Autodesk Fusion 360 part; units mm, degrees
(part 2 of 6)
  spline S10 degree 5 poles (8.3108, -19.4412) (8.3159, -19.4531) (8.3264, -19.4767) (8.3432, -19.5116) (8.3675, -19.5571) (8.4005, -19.6127) (8.4354, -19.6674) (8.4715, -19.7215) (8.5082, -19.7752) (8.5453, -19.8288) (8.583, -19.8822) (8.6212, -19.9352) (8.6602, -19.9878) (8.7001, -20.0399) (8.7409, -20.0915) (8.7826, -20.1426) (8.825, -20.1933) (8.868, -20.2437) (8.9115, -20.2938) (8.9555, -20.3436) (9, -20.3931) (9.045, -20.4423) (9.0905, -20.4911) (9.1367, -20.5396) (9.1833, -20.5878) (9.2305, -20.6356) (9.2782, -20.6831) (9.3264, -20.7304) (9.375, -20.7773) (9.424, -20.8239) (9.4735, -20.8702) (9.5235, -20.9163) (9.5738, -20.962) (9.6246, -21.0074) (9.6759, -21.0526) (9.7275, -21.0974) (9.7796, -21.142) (9.8321, -21.1862) (9.885, -21.2302) (9.9382, -21.2739) (9.9919, -21.3173) (10.0459, -21.3605) (10.1003, -21.4033) (10.155, -21.4459) (10.2102, -21.4882) (10.2657, -21.5302) (10.3216, -21.5719) (10.3778, -21.6133) (10.4343, -21.6545) (10.4913, -21.6954) (10.5485, -21.736) (10.6061, -21.7763) (10.664, -21.8163) (10.7223, -21.8561) (10.7809, -21.8956) (10.8398, -21.9348) (10.899, -21.9738) (10.9586, -22.0124) (11.0184, -22.0508) (11.0786, -22.0889) (11.1391, -22.1268) (11.1999, -22.1643) (11.261, -22.2016) (11.3224, -22.2386) (11.3841, -22.2754) (11.4461, -22.3119) (11.5083, -22.348) (11.5709, -22.384) (11.6337, -22.4196) (11.6969, -22.455) (11.7603, -22.4901) (11.8112, -22.5179) (11.8496, -22.5387) (11.8752, -22.5525) (11.888, -22.5594) knots 0 0 0 0 0 0 0.01428571 0.02857143 0.04285714 0.05714286 0.07142857 0.08571429 0.1 0.11428571 0.12857143 0.14285714 0.15714286 0.17142857 0.18571429 0.2 0.21428571 0.22857143 0.24285714 0.25714286 0.27142857 0.28571429 0.3 0.31428571 0.32857143 0.34285714 0.35714286 0.37142857 0.38571429 0.4 0.41428571 0.42857143 0.44285714 0.45714286 0.47142857 0.48571429 0.5 0.51428571 0.52857143 0.54285714 0.55714286 0.57142857 0.58571429 0.6 0.61428571 0.62857143 0.64285714 0.65714286 0.67142857 0.68571429 0.7 0.71428571 0.72857143 0.74285714 0.75714286 0.77142857 0.78571429 0.8 0.81428571 0.82857143 0.84285714 0.85714286 0.87142857 0.88571429 0.9 0.91428571 0.92857143 0.94285714 0.95714286 0.97142857 0.98571429 1 1 1 1 1 1
  arc A22 (11.888, -22.5594) -> (13.593, -21.575) centre (0, 0) ccw
  spline S11 degree 5 poles (13.593, -21.575) (13.5934, -21.5605) (13.5943, -21.5314) (13.5955, -21.4878) (13.5968, -21.4297) (13.5981, -21.3573) (13.5991, -21.2849) (13.5996, -21.2127) (13.5998, -21.1405) (13.5996, -21.0685) (13.599, -20.9966) (13.598, -20.9248) (13.5967, -20.8531) (13.5949, -20.7816) (13.5928, -20.7101) (13.5903, -20.6388) (13.5874, -20.5677) (13.584, -20.4966) (13.5803, -20.4257) (13.5762, -20.3549) (13.5717, -20.2843) (13.5668, -20.2138) (13.5615, -20.1435) (13.5558, -20.0733) (13.5496, -20.0033) (13.5431, -19.9334) (13.5362, -19.8636) (13.5288, -19.7941) (13.521, -19.7247) (13.5128, -19.6554) (13.5042, -19.5864) (13.4952, -19.5175) (13.4857, -19.4488) (13.4758, -19.3802) (13.4654, -19.3119) (13.4547, -19.2437) (13.4434, -19.1757) (13.4318, -19.108) (13.4197, -19.0404) (13.4071, -18.973) (13.3941, -18.9059) (13.3807, -18.8389) (13.3667, -18.7722) (13.3523, -18.7057) (13.3374, -18.6394) (13.322, -18.5734) (13.3062, -18.5076) (13.2898, -18.442) (13.273, -18.3767) (13.2557, -18.3117) (13.2379, -18.2469) (13.2195, -18.1824) (13.2006, -18.1182) (13.181, -18.0543) (13.1609, -17.9908) (13.1403, -17.9275) (13.1192, -17.8645) (13.0976, -17.8018) (13.0754, -17.7393) (13.0527, -17.6773) (13.0293, -17.6156) (13.005, -17.5545) (12.9798, -17.4938) (12.9538, -17.4338) (12.927, -17.3741) (12.8996, -17.3149) (12.8718, -17.2559) (12.8435, -17.1973) (12.8147, -17.139) (12.7848, -17.0814) (12.7532, -17.025) (12.7259, -16.9812) (12.7041, -16.9492) (12.6889, -16.9283) (12.6811, -16.918) knots -1 -1 -1 -1 -1 -1 -0.98571429 -0.97142857 -0.95714286 -0.94285714 -0.92857143 -0.91428571 -0.9 -0.88571429 -0.87142857 -0.85714286 -0.84285714 -0.82857143 -0.81428571 -0.8 -0.78571429 -0.77142857 -0.75714286 -0.74285714 -0.72857143 -0.71428571 -0.7 -0.68571429 -0.67142857 -0.65714286 -0.64285714 -0.62857143 -0.61428571 -0.6 -0.58571429 -0.57142857 -0.55714286 -0.54285714 -0.52857143 -0.51428571 -0.5 -0.48571429 -0.47142857 -0.45714286 -0.44285714 -0.42857143 -0.41428571 -0.4 -0.38571429 -0.37142857 -0.35714286 -0.34285714 -0.32857143 -0.31428571 -0.3 -0.28571429 -0.27142857 -0.25714286 -0.24285714 -0.22857143 -0.21428571 -0.2 -0.18571429 -0.17142857 -0.15714286 -0.14285714 -0.12857143 -0.11428571 -0.1 -0.08571429 -0.07142857 -0.05714286 -0.04285714 -0.02857143 -0.01428571 0 0 0 0 0 0
  line L11 (12.6811, -16.918) -> (12.1717, -16.2376)
  arc A23 (12.3867, -14.2079) -> (12.1717, -16.2376) centre (13.3724, -15.3385) ccw
  arc A24 (12.3867, -14.2079) -> (12.8353, -13.8039) centre (0, 0) ccw
  arc A25 (14.8763, -13.8023) -> (12.8353, -13.8039) centre (13.8567, -14.9024) ccw
  line L12 (14.8763, -13.8023) -> (15.4998, -14.3801)
  spline S12 degree 5 poles (15.4998, -14.3801) (15.5093, -14.3889) (15.5285, -14.4062) (15.558, -14.4312) (15.5987, -14.4629) (15.6515, -14.5003) (15.7056, -14.536) (15.7605, -14.5708) (15.8159, -14.605) (15.8717, -14.6388) (15.9277, -14.6723) (15.9842, -14.7051) (16.0412, -14.7373) (16.0989, -14.7687) (16.1572, -14.7992) (16.2161, -14.829) (16.2754, -14.8581) (16.3352, -14.8866) (16.3953, -14.9147) (16.4557, -14.9423) (16.5165, -14.9694) (16.5776, -14.996) (16.6391, -15.0221) (16.701, -15.0477) (16.7632, -15.0727) (16.8258, -15.0972) (16.8886, -15.1212) (16.9518, -15.1447) (17.0153, -15.1678) (17.0791, -15.1905) (17.1432, -15.2127) (17.2075, -15.2344) (17.2721, -15.2557) (17.337, -15.2766) (17.4022, -15.297) (17.4676, -15.3169) (17.5333, -15.3364) (17.5993, -15.3555) (17.6655, -15.3742) (17.7319, -15.3925) (17.7986, -15.4103) (17.8655, -15.4277) (17.9326, -15.4448) (17.9999, -15.4614) (18.0675, -15.4776) (18.1353, -15.4934) (18.2033, -15.5087) (18.2715, -15.5237) (18.3399, -15.5383) (18.4085, -15.5525) (18.4774, -15.5663) (18.5464, -15.5797) (18.6156, -15.5928) (18.685, -15.6054) (18.7546, -15.6177) (18.8243, -15.6295) (18.8943, -15.641) (18.9644, -15.6521) (19.0347, -15.6628) (19.1052, -15.6732) (19.1758, -15.6831) (19.2467, -15.6927) (19.3176, -15.7019) (19.3888, -15.7108) (19.4601, -15.7193) (19.5315, -15.7274) (19.6032, -15.7351) (19.6749, -15.7425) (19.7468, -15.7495) (19.8189, -15.7561) (19.8911, -15.7624) (19.949, -15.7671) (19.9924, -15.7705) (20.0215, -15.7726) (20.036, -15.7737) knots 0 0 0 0 0 0 0.01428571 0.02857143 0.04285714 0.05714286 0.07142857 0.08571429 0.1 0.11428571 0.12857143 0.14285714 0.15714286 0.17142857 0.18571429 0.2 0.21428571 0.22857143 0.24285714 0.25714286 0.27142857 0.28571429 0.3 0.31428571 0.32857143 0.34285714 0.35714286 0.37142857 0.38571429 0.4 0.41428571 0.42857143 0.44285714 0.45714286 0.47142857 0.48571429 0.5 0.51428571 0.52857143 0.54285714 0.55714286 0.57142857 0.58571429 0.6 0.61428571 0.62857143 0.64285714 0.65714286 0.67142857 0.68571429 0.7 0.71428571 0.72857143 0.74285714 0.75714286 0.77142857 0.78571429 0.8 0.81428571 0.82857143 0.84285714 0.85714286 0.87142857 0.88571429 0.9 0.91428571 0.92857143 0.94285714 0.95714286 0.97142857 0.98571429 1 1 1 1 1 1
  arc A26 (20.036, -15.7737) -> (21.1931, -14.181) centre (0, 0) ccw
  spline S13 degree 5 poles (21.1931, -14.181) (21.1876, -14.1675) (21.1766, -14.1406) (21.16, -14.1003) (21.1376, -14.0467) (21.1093, -13.98) (21.0807, -13.9135) (21.0519, -13.8473) (21.0227, -13.7813) (20.9932, -13.7156) (20.9634, -13.6501) (20.9333, -13.5849) (20.9029, -13.52) (20.8722, -13.4553) (20.8412, -13.391) (20.8099, -13.3268) (20.7783, -13.263) (20.7464, -13.1995) (20.7141, -13.1362) (20.6816, -13.0732) (20.6488, -13.0105) (20.6156, -12.9481) (20.5821, -12.886) (20.5484, -12.8242) (20.5143, -12.7627) (20.4799, -12.7016) (20.4452, -12.6407) (20.4101, -12.5801) (20.3748, -12.5199) (20.3392, -12.46) (20.3032, -12.4004) (20.2669, -12.3411) (20.2303, -12.2822) (20.1934, -12.2236) (20.1561, -12.1654) (20.1186, -12.1075) (20.0807, -12.05) (20.0425, -11.9928) (20.0039, -11.936) (19.965, -11.8795) (19.9258, -11.8235) (19.8863, -11.7678) (19.8464, -11.7125) (19.8062, -11.6576) (19.7656, -11.6032) (19.7247, -11.5491) (19.6835, -11.4954) (19.6419, -11.4422) (19.6, -11.3893) (19.5577, -11.337) (19.5151, -11.285) (19.4721, -11.2336) (19.4286, -11.1826) (19.3848, -11.1322) (19.3406, -11.0823) (19.2961, -11.0329) (19.2511, -10.984) (19.2059, -10.9355) (19.1603, -10.8874) (19.1142, -10.84) (19.0677, -10.7932) (19.0207, -10.7472) (18.973, -10.702) (18.9248, -10.6577) (18.8761, -10.6142) (18.827, -10.5712) (18.7776, -10.5287) (18.7279, -10.4865) (18.6779, -10.445) (18.6272, -10.4046) (18.5753, -10.366) (18.5326, -10.337) (18.4996, -10.3167) (18.4773, -10.3038) (18.466, -10.2975) knots -1 -1 -1 -1 -1 -1 -0.98571429 -0.97142857 -0.95714286 -0.94285714 -0.92857143 -0.91428571 -0.9 -0.88571429 -0.87142857 -0.85714286 -0.84285714 -0.82857143 -0.81428571 -0.8 -0.78571429 -0.77142857 -0.75714286 -0.74285714 -0.72857143 -0.71428571 -0.7 -0.68571429 -0.67142857 -0.65714286 -0.64285714 -0.62857143 -0.61428571 -0.6 -0.58571429 -0.57142857 -0.55714286 -0.54285714 -0.52857143 -0.51428571 -0.5 -0.48571429 -0.47142857 -0.45714286 -0.44285714 -0.42857143 -0.41428571 -0.4 -0.38571429 -0.37142857 -0.35714286 -0.34285714 -0.32857143 -0.31428571 -0.3 -0.28571429 -0.27142857 -0.25714286 -0.24285714 -0.22857143 -0.21428571 -0.2 -0.18571429 -0.17142857 -0.15714286 -0.14285714 -0.12857143 -0.11428571 -0.1 -0.08571429 -0.07142857 -0.05714286 -0.04285714 -0.02857143 -0.01428571 0 0 0 0 0 0
  line L13 (18.466, -10.2975) -> (17.7238, -9.8831)
  arc A27 (17.0946, -7.9414) -> (17.7238, -9.8831) centre (18.455, -8.5734) ccw
  arc A28 (17.0946, -7.9414) -> (17.3402, -7.3899) centre (0, 0) ccw
  arc A29 (19.2041, -6.5583) -> (17.3402, -7.3899) centre (18.7201, -7.978) ccw
  line L14 (19.2041, -6.5583) -> (20.0087, -6.8325)
  spline S14 degree 5 poles (20.0087, -6.8325) (20.0209, -6.8367) (20.0455, -6.8447) (20.0826, -6.8556) (20.1327, -6.868) (20.1961, -6.8807) (20.2601, -6.8913) (20.3244, -6.9007) (20.389, -6.9094) (20.4536, -6.9176) (20.5184, -6.9254) (20.5834, -6.9325) (20.6486, -6.9387) (20.714, -6.9438) (20.7797, -6.948) (20.8456, -6.9513) (20.9117, -6.9537) (20.9779, -6.9555) (21.0442, -6.9567) (21.1106, -6.9573) (21.1772, -6.9574) (21.2438, -6.9568) (21.3106, -6.9556) (21.3775, -6.9538) (21.4445, -6.9514) (21.5117, -6.9483) (21.5789, -6.9447) (21.6462, -6.9405) (21.7136, -6.9357) (21.7811, -6.9305) (21.8486, -6.9247) (21.9163, -6.9184) (21.9839, -6.9116) (22.0517, -6.9042) (22.1195, -6.8963) (22.1874, -6.888) (22.2554, -6.8791) (22.3234, -6.8697) (22.3915, -6.8598) (22.4596, -6.8495) (22.5277, -6.8387) (22.5959, -6.8274) (22.6642, -6.8157) (22.7324, -6.8034) (22.8008, -6.7907) (22.8691, -6.7776) (22.9375, -6.764) (23.0059, -6.7499) (23.0744, -6.7355) (23.1428, -6.7205) (23.2113, -6.7051) (23.2798, -6.6893) (23.3483, -6.6731) (23.4169, -6.6564) (23.4854, -6.6393) (23.554, -6.6217) (23.6226, -6.6038) (23.6911, -6.5854) (23.7597, -6.5666) (23.8283, -6.5474) (23.8969, -6.5277) (23.9655, -6.5077) (24.0341, -6.4873) (24.1027, -6.4664) (24.1713, -6.4451) (24.2398, -6.4235) (24.3084, -6.4014) (24.377, -6.3789) (24.4455, -6.3561) (24.514, -6.3328) (24.5825, -6.3092) (24.6373, -6.29) (24.6784, -6.2754) (24.7058, -6.2656) (24.7195, -6.2606) knots 0 0 0 0 0 0 0.01428571 0.02857143 0.04285714 0.05714286 0.07142857 0.08571429 0.1 0.11428571 0.12857143 0.14285714 0.15714286 0.17142857 0.18571429 0.2 0.21428571 0.22857143 0.24285714 0.25714286 0.27142857 0.28571429 0.3 0.31428571 0.32857143 0.34285714 0.35714286 0.37142857 0.38571429 0.4 0.41428571 0.42857143 0.44285714 0.45714286 0.47142857 0.48571429 0.5 0.51428571 0.52857143 0.54285714 0.55714286 0.57142857 0.58571429 0.6 0.61428571 0.62857143 0.64285714 0.65714286 0.67142857 0.68571429 0.7 0.71428571 0.72857143 0.74285714 0.75714286 0.77142857 0.78571429 0.8 0.81428571 0.82857143 0.84285714 0.85714286 0.87142857 0.88571429 0.9 0.91428571 0.92857143 0.94285714 0.95714286 0.97142857 0.98571429 1 1 1 1 1 1
  arc A30 (24.7195, -6.2606) -> (25.1288, -4.335) centre (0, 0) ccw
  spline S15 degree 5 poles (25.1288, -4.335) (25.1183, -4.3249) (25.0973, -4.3048) (25.0657, -4.2747) (25.0234, -4.2349) (24.9705, -4.1854) (24.9173, -4.1363) (24.864, -4.0875) (24.8105, -4.0391) (24.7569, -3.9911) (24.703, -3.9434) (24.649, -3.8961) (24.5948, -3.8491) (24.5405, -3.8026) (24.486, -3.7564) (24.4313, -3.7105) (24.3765, -3.6651) (24.3215, -3.62) (24.2663, -3.5753) (24.2109, -3.531) (24.1554, -3.4871) (24.0998, -3.4436) (24.0439, -3.4005) (23.9879, -3.3578) (23.9318, -3.3154) (23.8755, -3.2735) (23.819, -3.232) (23.7624, -3.191) (23.7056, -3.1503) (23.6487, -3.1101) (23.5916, -3.0703) (23.5343, -3.0309) (23.4769, -2.9919) (23.4194, -2.9534) (23.3617, -2.9154) (23.3038, -2.8778) (23.2458, -2.8406) (23.1876, -2.804) (23.1293, -2.7677) (23.0708, -2.732) (23.0122, -2.6967) (22.9534, -2.6619) (22.8945, -2.6276) (22.8355, -2.5939) (22.7762, -2.5606) (22.7169, -2.5278) (22.6574, -2.4956) (22.5977, -2.4639) (22.538, -2.4326) (22.478, -2.402) (22.4179, -2.3719) (22.3577, -2.3424) (22.2973, -2.3135) (22.2368, -2.2853) (22.1761, -2.2577) (22.1153, -2.2307) (22.0544, -2.2042) (21.9933, -2.1783) (21.9321, -2.153) (21.8707, -2.1284) (21.8092, -2.1045) (21.7475, -2.0816) (21.6856, -2.0598) (21.6236, -2.0389) (21.5613, -2.019) (21.499, -1.9997) (21.4366, -1.9809) (21.3741, -1.9626) (21.3115, -1.945) (21.2487, -1.9287) (21.1856, -1.9145) (21.1348, -1.9055) (21.0964, -1.9003) (21.0707, -1.8976) (21.0579, -1.8964) knots -1 -1 -1 -1 -1 -1 -0.98571429 -0.97142857 -0.95714286 -0.94285714 -0.92857143 -0.91428571 -0.9 -0.88571429 -0.87142857 -0.85714286 -0.84285714 -0.82857143 -0.81428571 -0.8 -0.78571429 -0.77142857 -0.75714286 -0.74285714 -0.72857143 -0.71428571 -0.7 -0.68571429 -0.67142857 -0.65714286 -0.64285714 -0.62857143 -0.61428571 -0.6 -0.58571429 -0.57142857 -0.55714286 -0.54285714 -0.52857143 -0.51428571 -0.5 -0.48571429 -0.47142857 -0.45714286 -0.44285714 -0.42857143 -0.41428571 -0.4 -0.38571429 -0.37142857 -0.35714286 -0.34285714 -0.32857143 -0.31428571 -0.3 -0.28571429 -0.27142857 -0.25714286 -0.24285714 -0.22857143 -0.21428571 -0.2 -0.18571429 -0.17142857 -0.15714286 -0.14285714 -0.12857143 -0.11428571 -0.1 -0.08571429 -0.07142857 -0.05714286 -0.04285714 -0.02857143 -0.01428571 0 0 0 0 0 0
  line L15 (21.0579, -1.8964) -> (20.2113, -1.8197)
  arc A31 (18.8468, -0.3018) -> (20.2113, -1.8197) centre (20.3466, -0.3259) ccw
  arc A32 (18.8468, -0.3018) -> (18.8468, 0.3018) centre (0, 0) ccw
  arc A33 (20.2113, 1.8197) -> (18.8468, 0.3018) centre (20.3466, 0.3259) ccw
  line L16 (20.2113, 1.8197) -> (21.0579, 1.8964)
  spline S16 degree 5 poles (21.0579, 1.8964) (21.0707, 1.8976) (21.0964, 1.9003) (21.1348, 1.9055) (21.1856, 1.9145) (21.2487, 1.9287) (21.3115, 1.945) (21.3741, 1.9626) (21.4366, 1.9809) (21.499, 1.9997) (21.5613, 2.019) (21.6236, 2.0389) (21.6856, 2.0598) (21.7475, 2.0816) (21.8092, 2.1045) (21.8707, 2.1284) (21.9321, 2.153) (21.9933, 2.1783) (22.0544, 2.2042) (22.1153, 2.2307) (22.1761, 2.2577) (22.2368, 2.2853) (22.2973, 2.3135) (22.3577, 2.3424) (22.4179, 2.3719) (22.478, 2.402) (22.538, 2.4326) (22.5977, 2.4639) (22.6574, 2.4956) (22.7169, 2.5278) (22.7762, 2.5606) (22.8355, 2.5939) (22.8945, 2.6276) (22.9534, 2.6619) (23.0122, 2.6967) (23.0708, 2.732) (23.1293, 2.7677) (23.1876, 2.804) (23.2458, 2.8406) (23.3038, 2.8778) (23.3617, 2.9154) (23.4194, 2.9534) (23.4769, 2.9919) (23.5343, 3.0309) (23.5916, 3.0703) (23.6487, 3.1101) (23.7056, 3.1503) (23.7624, 3.191) (23.819, 3.232) (23.8755, 3.2735) (23.9318, 3.3154) (23.9879, 3.3578) (24.0439, 3.4005) (24.0998, 3.4436) (24.1554, 3.4871) (24.2109, 3.531) (24.2663, 3.5753) (24.3215, 3.62) (24.3765, 3.6651) (24.4313, 3.7105) (24.486, 3.7564) (24.5405, 3.8026) (24.5948, 3.8491) (24.649, 3.8961) (24.703, 3.9434) (24.7569, 3.9911) (24.8105, 4.0391) (24.864, 4.0875) (24.9173, 4.1363) (24.9705, 4.1854) (25.0234, 4.2349) (25.0657, 4.2747) (25.0973, 4.3048) (25.1183, 4.3249) (25.1288, 4.335) knots 0 0 0 0 0 0 0.01428571 0.02857143 0.04285714 0.05714286 0.07142857 0.08571429 0.1 0.11428571 0.12857143 0.14285714 0.15714286 0.17142857 0.18571429 0.2 0.21428571 0.22857143 0.24285714 0.25714286 0.27142857 0.28571429 0.3 0.31428571 0.32857143 0.34285714 0.35714286 0.37142857 0.38571429 0.4 0.41428571 0.42857143 0.44285714 0.45714286 0.47142857 0.48571429 0.5 0.51428571 0.52857143 0.54285714 0.55714286 0.57142857 0.58571429 0.6 0.61428571 0.62857143 0.64285714 0.65714286 0.67142857 0.68571429 0.7 0.71428571 0.72857143 0.74285714 0.75714286 0.77142857 0.78571429 0.8 0.81428571 0.82857143 0.84285714 0.85714286 0.87142857 0.88571429 0.9 0.91428571 0.92857143 0.94285714 0.95714286 0.97142857 0.98571429 1 1 1 1 1 1
  arc A34 (25.1288, 4.335) -> (24.7195, 6.2606) centre (0, 0) ccw
  spline S17 degree 5 poles (24.7195, 6.2606) (24.7058, 6.2656) (24.6784, 6.2754) (24.6373, 6.29) (24.5825, 6.3092) (24.514, 6.3328) (24.4455, 6.3561) (24.377, 6.3789) (24.3084, 6.4014) (24.2398, 6.4235) (24.1713, 6.4451) (24.1027, 6.4664) (24.0341, 6.4873) (23.9655, 6.5077) (23.8969, 6.5277) (23.8283, 6.5474) (23.7597, 6.5666) (23.6911, 6.5854) (23.6226, 6.6038) (23.554, 6.6217) (23.4854, 6.6393) (23.4169, 6.6564) (23.3483, 6.6731) (23.2798, 6.6893) (23.2113, 6.7051) (23.1428, 6.7205) (23.0744, 6.7355) (23.0059, 6.7499) (22.9375, 6.764) (22.8691, 6.7776) (22.8008, 6.7907) (22.7324, 6.8034) (22.6642, 6.8157) (22.5959, 6.8274) (22.5277, 6.8387) (22.4596, 6.8495) (22.3915, 6.8598) (22.3234, 6.8697) (22.2554, 6.8791) (22.1874, 6.888) (22.1195, 6.8963) (22.0517, 6.9042) (21.9839, 6.9116) (21.9163, 6.9184) (21.8486, 6.9247) (21.7811, 6.9305) (21.7136, 6.9357) (21.6462, 6.9405) (21.5789, 6.9447) (21.5117, 6.9483) (21.4445, 6.9514) (21.3775, 6.9538) (21.3106, 6.9556) (21.2438, 6.9568) (21.1772, 6.9574) (21.1106, 6.9573) (21.0442, 6.9567) (20.9779, 6.9555) (20.9117, 6.9537) (20.8456, 6.9513) (20.7797, 6.948) (20.714, 6.9438) (20.6486, 6.9387) (20.5834, 6.9325) (20.5184, 6.9254) (20.4536, 6.9176) (20.389, 6.9094) (20.3244, 6.9007) (20.2601, 6.8913) (20.1961, 6.8807) (20.1327, 6.868) (20.0826, 6.8556) (20.0455, 6.8447) (20.0209, 6.8367) (20.0087, 6.8325) knots -1 -1 -1 -1 -1 -1 -0.98571429 -0.97142857 -0.95714286 -0.94285714 -0.92857143 -0.91428571 -0.9 -0.88571429 -0.87142857 -0.85714286 -0.84285714 -0.82857143 -0.81428571 -0.8 -0.78571429 -0.77142857 -0.75714286 -0.74285714 -0.72857143 -0.71428571 -0.7 -0.68571429 -0.67142857 -0.65714286 -0.64285714 -0.62857143 -0.61428571 -0.6 -0.58571429 -0.57142857 -0.55714286 -0.54285714 -0.52857143 -0.51428571 -0.5 -0.48571429 -0.47142857 -0.45714286 -0.44285714 -0.42857143 -0.41428571 -0.4 -0.38571429 -0.37142857 -0.35714286 -0.34285714 -0.32857143 -0.31428571 -0.3 -0.28571429 -0.27142857 -0.25714286 -0.24285714 -0.22857143 -0.21428571 -0.2 -0.18571429 -0.17142857 -0.15714286 -0.14285714 -0.12857143 -0.11428571 -0.1 -0.08571429 -0.07142857 -0.05714286 -0.04285714 -0.02857143 -0.01428571 0 0 0 0 0 0
  line L17 (20.0087, 6.8325) -> (19.2041, 6.5583)
  arc A35 (17.3402, 7.3899) -> (19.2041, 6.5583) centre (18.7201, 7.978) ccw
  arc A36 (17.3402, 7.3899) -> (17.0946, 7.9414) centre (0, 0) ccw
  arc A37 (17.7238, 9.8831) -> (17.0946, 7.9414) centre (18.455, 8.5734) ccw
  line L18 (17.7238, 9.8831) -> (18.466, 10.2975)
  spline S18 degree 5 poles (18.466, 10.2975) (18.4773, 10.3038) (18.4996, 10.3167) (18.5326, 10.337) (18.5753, 10.366) (18.6272, 10.4046) (18.6779, 10.445) (18.7279, 10.4865) (18.7776, 10.5287) (18.827, 10.5712) (18.8761, 10.6142) (18.9248, 10.6577) (18.973, 10.702) (19.0207, 10.7472) (19.0677, 10.7932) (19.1142, 10.84) (19.1603, 10.8874) (19.2059, 10.9355) (19.2511, 10.984) (19.2961, 11.0329) (19.3406, 11.0823) (19.3848, 11.1322) (19.4286, 11.1826) (19.4721, 11.2336) (19.5151, 11.285) (19.5577, 11.337) (19.6, 11.3893) (19.6419, 11.4422) (19.6835, 11.4954) (19.7247, 11.5491) (19.7656, 11.6032) (19.8062, 11.6576) (19.8464, 11.7125) (19.8863, 11.7678) (19.9258, 11.8235) (19.965, 11.8795) (20.0039, 11.936) (20.0425, 11.9928) (20.0807, 12.05) (20.1186, 12.1075) (20.1561, 12.1654) (20.1934, 12.2236) (20.2303, 12.2822) (20.2669, 12.3411) (20.3032, 12.4004) (20.3392, 12.46) (20.3748, 12.5199) (20.4101, 12.5801) (20.4452, 12.6407) (20.4799, 12.7016) (20.5143, 12.7627) (20.5484, 12.8242) (20.5821, 12.886) (20.6156, 12.9481) (20.6488, 13.0105) (20.6816, 13.0732) (20.7141, 13.1362) (20.7464, 13.1995) (20.7783, 13.263) (20.8099, 13.3268) (20.8412, 13.391) (20.8722, 13.4553) (20.9029, 13.52) (20.9333, 13.5849) (20.9634, 13.6501) (20.9932, 13.7156) (21.0227, 13.7813) (21.0519, 13.8473) (21.0807, 13.9135) (21.1093, 13.98) (21.1376, 14.0467) (21.16, 14.1003) (21.1766, 14.1406) (21.1876, 14.1675) (21.1931, 14.181) knots 0 0 0 0 0 0 0.01428571 0.02857143 0.04285714 0.05714286 0.07142857 0.08571429 0.1 0.11428571 0.12857143 0.14285714 0.15714286 0.17142857 0.18571429 0.2 0.21428571 0.22857143 0.24285714 0.25714286 0.27142857 0.28571429 0.3 0.31428571 0.32857143 0.34285714 0.35714286 0.37142857 0.38571429 0.4 0.41428571 0.42857143 0.44285714 0.45714286 0.47142857 0.48571429 0.5 0.51428571 0.52857143 0.54285714 0.55714286 0.57142857 0.58571429 0.6 0.61428571 0.62857143 0.64285714 0.65714286 0.67142857 0.68571429 0.7 0.71428571 0.72857143 0.74285714 0.75714286 0.77142857 0.78571429 0.8 0.81428571 0.82857143 0.84285714 0.85714286 0.87142857 0.88571429 0.9 0.91428571 0.92857143 0.94285714 0.95714286 0.97142857 0.98571429 1 1 1 1 1 1
  arc A38 (21.1931, 14.181) -> (20.036, 15.7737) centre (0, 0) ccw
  spline S19 degree 5 poles (20.036, 15.7737) (20.0215, 15.7726) (19.9924, 15.7705) (19.949, 15.7671) (19.8911, 15.7624) (19.8189, 15.7561) (19.7468, 15.7495) (19.6749, 15.7425) (19.6032, 15.7351) (19.5315, 15.7274) (19.4601, 15.7193) (19.3888, 15.7108) (19.3176, 15.7019) (19.2467, 15.6927) (19.1758, 15.6831) (19.1052, 15.6732) (19.0347, 15.6628) (18.9644, 15.6521) (18.8943, 15.641) (18.8243, 15.6295) (18.7546, 15.6177) (18.685, 15.6054) (18.6156, 15.5928) (18.5464, 15.5797) (18.4774, 15.5663) (18.4085, 15.5525) (18.3399, 15.5383) (18.2715, 15.5237) (18.2033, 15.5087) (18.1353, 15.4934) (18.0675, 15.4776) (17.9999, 15.4614) (17.9326, 15.4448) (17.8655, 15.4277) (17.7986, 15.4103) (17.7319, 15.3925) (17.6655, 15.3742) (17.5993, 15.3555) (17.5333, 15.3364) (17.4676, 15.3169) (17.4022, 15.297) (17.337, 15.2766) (17.2721, 15.2557) (17.2075, 15.2344) (17.1432, 15.2127) (17.0791, 15.1905) (17.0153, 15.1678) (16.9518, 15.1447) (16.8886, 15.1212) (16.8258, 15.0972) (16.7632, 15.0727) (16.701, 15.0477) (16.6391, 15.0221) (16.5776, 14.996) (16.5165, 14.9694) (16.4557, 14.9423) (16.3953, 14.9147) (16.3352, 14.8866) (16.2754, 14.8581) (16.2161, 14.829) (16.1572, 14.7992) (16.0989, 14.7687) (16.0412, 14.7373) (15.9842, 14.7051) (15.9277, 14.6723) (15.8717, 14.6388) (15.8159, 14.605) (15.7605, 14.5708) (15.7056, 14.536) (15.6515, 14.5003) (15.5987, 14.4629) (15.558, 14.4312) (15.5285, 14.4062) (15.5093, 14.3889) (15.4998, 14.3801) knots -1 -1 -1 -1 -1 -1 -0.98571429 -0.97142857 -0.95714286 -0.94285714 -0.92857143 -0.91428571 -0.9 -0.88571429 -0.87142857 -0.85714286 -0.84285714 -0.82857143 -0.81428571 -0.8 -0.78571429 -0.77142857 -0.75714286 -0.74285714 -0.72857143 -0.71428571 -0.7 -0.68571429 -0.67142857 -0.65714286 -0.64285714 -0.62857143 -0.61428571 -0.6 -0.58571429 -0.57142857 -0.55714286 -0.54285714 -0.52857143 -0.51428571 -0.5 -0.48571429 -0.47142857 -0.45714286 -0.44285714 -0.42857143 -0.41428571 -0.4 -0.38571429 -0.37142857 -0.35714286 -0.34285714 -0.32857143 -0.31428571 -0.3 -0.28571429 -0.27142857 -0.25714286 -0.24285714 -0.22857143 -0.21428571 -0.2 -0.18571429 -0.17142857 -0.15714286 -0.14285714 -0.12857143 -0.11428571 -0.1 -0.08571429 -0.07142857 -0.05714286 -0.04285714 -0.02857143 -0.01428571 0 0 0 0 0 0
  line L19 (15.4998, 14.3801) -> (14.8763, 13.8023)
  arc A39 (12.8353, 13.8039) -> (14.8763, 13.8023) centre (13.8567, 14.9024) ccw
  arc A40 (12.8353, 13.8039) -> (12.3867, 14.2079) centre (0, 0) ccw
  arc A41 (12.1717, 16.2376) -> (12.3867, 14.2079) centre (13.3724, 15.3385) ccw
  line L20 (12.1717, 16.2376) -> (12.6811, 16.918)
  spline S20 degree 5 poles (12.6811, 16.918) (12.6889, 16.9283) (12.7041, 16.9492) (12.7259, 16.9812) (12.7532, 17.025) (12.7848, 17.0814) (12.8147, 17.139) (12.8435, 17.1973) (12.8718, 17.2559) (12.8996, 17.3149) (12.927, 17.3741) (12.9538, 17.4338) (12.9798, 17.4938) (13.005, 17.5545) (13.0293, 17.6156) (13.0527, 17.6773) (13.0754, 17.7393) (13.0976, 17.8018) (13.1192, 17.8645) (13.1403, 17.9275) (13.1609, 17.9908) (13.181, 18.0543) (13.2006, 18.1182) (13.2195, 18.1824) (13.2379, 18.2469) (13.2557, 18.3117) (13.273, 18.3767) (13.2898, 18.442) (13.3062, 18.5076) (13.322, 18.5734) (13.3374, 18.6394) (13.3523, 18.7057) (13.3667, 18.7722) (13.3807, 18.8389) (13.3941, 18.9059) (13.4071, 18.973) (13.4197, 19.0404) (13.4318, 19.108) (13.4434, 19.1757) (13.4547, 19.2437) (13.4654, 19.3119) (13.4758, 19.3802) (13.4857, 19.4488) (13.4952, 19.5175) (13.5042, 19.5864) (13.5128, 19.6554) (13.521, 19.7247) (13.5288, 19.7941) (13.5362, 19.8636) (13.5431, 19.9334) (13.5496, 20.0033) (13.5558, 20.0733) (13.5615, 20.1435) (13.5668, 20.2138) (13.5717, 20.2843) (13.5762, 20.3549) (13.5803, 20.4257) (13.584, 20.4966) (13.5874, 20.5677) (13.5903, 20.6388) (13.5928, 20.7101) (13.5949, 20.7816) (13.5967, 20.8531) (13.598, 20.9248) (13.599, 20.9966) (13.5996, 21.0685) (13.5998, 21.1405) (13.5996, 21.2127) (13.5991, 21.2849) (13.5981, 21.3573) (13.5968, 21.4297) (13.5955, 21.4878) (13.5943, 21.5314) (13.5934, 21.5605) (13.593, 21.575) knots 0 0 0 0 0 0 0.01428571 0.02857143 0.04285714 0.05714286 0.07142857 0.08571429 0.1 0.11428571 0.12857143 0.14285714 0.15714286 0.17142857 0.18571429 0.2 0.21428571 0.22857143 0.24285714 0.25714286 0.27142857 0.28571429 0.3 0.31428571 0.32857143 0.34285714 0.35714286 0.37142857 0.38571429 0.4 0.41428571 0.42857143 0.44285714 0.45714286 0.47142857 0.48571429 0.5 0.51428571 0.52857143 0.54285714 0.55714286 0.57142857 0.58571429 0.6 0.61428571 0.62857143 0.64285714 0.65714286 0.67142857 0.68571429 0.7 0.71428571 0.72857143 0.74285714 0.75714286 0.77142857 0.78571429 0.8 0.81428571 0.82857143 0.84285714 0.85714286 0.87142857 0.88571429 0.9 0.91428571 0.92857143 0.94285714 0.95714286 0.97142857 0.98571429 1 1 1 1 1 1
  arc A42 (13.593, 21.575) -> (11.888, 22.5594) centre (0, 0) ccw
  spline S21 degree 5 poles (11.888, 22.5594) (11.8752, 22.5525) (11.8496, 22.5387) (11.8112, 22.5179) (11.7603, 22.4901) (11.6969, 22.455) (11.6337, 22.4196) (11.5709, 22.384) (11.5083, 22.348) (11.4461, 22.3119) (11.3841, 22.2754) (11.3224, 22.2386) (11.261, 22.2016) (11.1999, 22.1643) (11.1391, 22.1268) (11.0786, 22.0889) (11.0184, 22.0508) (10.9586, 22.0124) (10.899, 21.9738) (10.8398, 21.9348) (10.7809, 21.8956) (10.7223, 21.8561) (10.664, 21.8163) (10.6061, 21.7763) (10.5485, 21.736) (10.4913, 21.6954) (10.4343, 21.6545) (10.3778, 21.6133) (10.3216, 21.5719) (10.2657, 21.5302) (10.2102, 21.4882) (10.155, 21.4459) (10.1003, 21.4033) (10.0459, 21.3605) (9.9919, 21.3173) (9.9382, 21.2739) (9.885, 21.2302) (9.8321, 21.1862) (9.7796, 21.142) (9.7275, 21.0974) (9.6759, 21.0526) (9.6246, 21.0074) (9.5738, 20.962) (9.5235, 20.9163) (9.4735, 20.8702) (9.424, 20.8239) (9.375, 20.7773) (9.3264, 20.7304) (9.2782, 20.6831) (9.2305, 20.6356) (9.1833, 20.5878) (9.1367, 20.5396) (9.0905, 20.4911) (9.045, 20.4423) (9, 20.3931) (8.9555, 20.3436) (8.9115, 20.2938) (8.868, 20.2437) (8.825, 20.1933) (8.7826, 20.1426) (8.7409, 20.0915) (8.7001, 20.0399) (8.6602, 19.9878) (8.6212, 19.9352) (8.583, 19.8822) (8.5453, 19.8288) (8.5082, 19.7752) (8.4715, 19.7215) (8.4354, 19.6674) (8.4005, 19.6127) (8.3675, 19.5571) (8.3432, 19.5116) (8.3264, 19.4767) (8.3159, 19.4531) (8.3108, 19.4412) knots -1 -1 -1 -1 -1 -1 -0.98571429 -0.97142857 -0.95714286 -0.94285714 -0.92857143 -0.91428571 -0.9 -0.88571429 -0.87142857 -0.85714286 -0.84285714 -0.82857143 -0.81428571 -0.8 -0.78571429 -0.77142857 -0.75714286 -0.74285714 -0.72857143 -0.71428571 -0.7 -0.68571429 -0.67142857 -0.65714286 -0.64285714 -0.62857143 -0.61428571 -0.6 -0.58571429 -0.57142857 -0.55714286 -0.54285714 -0.52857143 -0.51428571 -0.5 -0.48571429 -0.47142857 -0.45714286 -0.44285714 -0.42857143 -0.41428571 -0.4 -0.38571429 -0.37142857 -0.35714286 -0.34285714 -0.32857143 -0.31428571 -0.3 -0.28571429 -0.27142857 -0.25714286 -0.24285714 -0.22857143 -0.21428571 -0.2 -0.18571429 -0.17142857 -0.15714286 -0.14285714 -0.12857143 -0.11428571 -0.1 -0.08571429 -0.07142857 -0.05714286 -0.04285714 -0.02857143 -0.01428571 0 0 0 0 0 0
  line L21 (8.3108, 19.4412) -> (7.9763, 18.6597)
  arc A43 (6.111, 17.8311) -> (7.9763, 18.6597) centre (6.5974, 19.2501) ccw
  arc A44 (6.111, 17.8311) -> (5.5369, 18.0176) centre (0, 0) ccw
  arc A45 (4.515, 19.7844) -> (5.5369, 18.0176) centre (5.9775, 19.4515) ccw
  line L22 (4.515, 19.7844) -> (4.7036, 20.6132)
  spline S22 degree 5 poles (4.7036, 20.6132) (4.7065, 20.6258) (4.7119, 20.6511) (4.7188, 20.6892) (4.7259, 20.7403) (4.7319, 20.8047) (4.7358, 20.8695) (4.7384, 20.9344) (4.7403, 20.9995) (4.7418, 21.0647) (4.7427, 21.1299) (4.7429, 21.1953) (4.7423, 21.2608) (4.7406, 21.3264) (4.7379, 21.3921) (4.7342, 21.458) (4.7298, 21.524) (4.7246, 21.59) (4.7188, 21.6561) (4.7125, 21.7222) (4.7056, 21.7884) (4.6981, 21.8547) (4.69, 21.9209) (4.6812, 21.9873) (4.6717, 22.0537) (4.6617, 22.1201) (4.651, 22.1866) (4.6398, 22.2531) (4.6281, 22.3196) (4.6158, 22.3862) (4.603, 22.4528) (4.5896, 22.5194) (4.5758, 22.586) (4.5614, 22.6526) (4.5464, 22.7192) (4.531, 22.7859) (4.5151, 22.8525) (4.4986, 22.9192) (4.4817, 22.9858) (4.4643, 23.0525) (4.4464, 23.1192) (4.4281, 23.1858) (4.4093, 23.2524) (4.39, 23.3191) (4.3702, 23.3857) (4.35, 23.4523) (4.3293, 23.5189) (4.3082, 23.5854) (4.2866, 23.652) (4.2646, 23.7185) (4.2422, 23.785) (4.2193, 23.8515) (4.1959, 23.9179) (4.1722, 23.9844) (4.148, 24.0508) (4.1234, 24.1171) (4.0984, 24.1834) (4.0729, 24.2497) (4.047, 24.316) (4.0208, 24.3822) (3.9941, 24.4483) (3.967, 24.5145) (3.9395, 24.5805) (3.9116, 24.6466) (3.8832, 24.7126) (3.8545, 24.7785) (3.8254, 24.8444) (3.7959, 24.9102) (3.766, 24.976) (3.7357, 25.0417) (3.7051, 25.1074) (3.6802, 25.1599) (3.6614, 25.1992) (3.6488, 25.2254) (3.6424, 25.2385) knots 0 0 0 0 0 0 0.01428571 0.02857143 0.04285714 0.05714286 0.07142857 0.08571429 0.1 0.11428571 0.12857143 0.14285714 0.15714286 0.17142857 0.18571429 0.2 0.21428571 0.22857143 0.24285714 0.25714286 0.27142857 0.28571429 0.3 0.31428571 0.32857143 0.34285714 0.35714286 0.37142857 0.38571429 0.4 0.41428571 0.42857143 0.44285714 0.45714286 0.47142857 0.48571429 0.5 0.51428571 0.52857143 0.54285714 0.55714286 0.57142857 0.58571429 0.6 0.61428571 0.62857143 0.64285714 0.65714286 0.67142857 0.68571429 0.7 0.71428571 0.72857143 0.74285714 0.75714286 0.77142857 0.78571429 0.8 0.81428571 0.82857143 0.84285714 0.85714286 0.87142857 0.88571429 0.9 0.91428571 0.92857143 0.94285714 0.95714286 0.97142857 0.98571429 1 1 1 1 1 1
  arc A46 (3.6424, 25.2385) -> (1.6845, 25.4443) centre (0, 0) ccw
  spline S23 degree 5 poles (1.6845, 25.4443) (1.6756, 25.4328) (1.6578, 25.4098) (1.6312, 25.3752) (1.596, 25.329) (1.5524, 25.2712) (1.5091, 25.2132) (1.4662, 25.1551) (1.4236, 25.0968) (1.3814, 25.0384) (1.3396, 24.9799) (1.2982, 24.9212) (1.2572, 24.8625) (1.2166, 24.8035) (1.1763, 24.7445) (1.1364, 24.6853) (1.097, 24.626) (1.0579, 24.5666) (1.0192, 24.5071) (0.9809, 24.4474) (0.9431, 24.3876) (0.9056, 24.3277) (0.8686, 24.2677) (0.8319, 24.2075) (0.7957, 24.1473) (0.7599, 24.0869) (0.7246, 24.0264) (0.6896, 23.9658) (0.6551, 23.905) (0.6211, 23.8442) (0.5874, 23.7833) (0.5543, 23.7222) (0.5215, 23.6611) (0.4893, 23.5998) (0.4575, 23.5384) (0.4261, 23.4769) (0.3952, 23.4154) (0.3648, 23.3537) (0.3349, 23.2919) (0.3055, 23.23) (0.2765, 23.168) (0.2481, 23.1059) (0.2201, 23.0438) (0.1927, 22.9815) (0.1658, 22.9191) (0.1394, 22.8567) (0.1136, 22.7941) (0.0883, 22.7315) (0.0635, 22.6688) (0.0392, 22.606) (0.0156, 22.5431) (-0.0075, 22.4801) (-0.0299, 22.417) (-0.0516, 22.3539) (-0.0727, 22.2906) (-0.0932, 22.2273) (-0.1132, 22.1639) (-0.1325, 22.1005) (-0.1513, 22.037) (-0.1694, 21.9734) (-0.1867, 21.9097) (-0.203, 21.846) (-0.2183, 21.7822) (-0.2325, 21.7182) (-0.2459, 21.6543) (-0.2585, 21.5902) (-0.2707, 21.5262) (-0.2824, 21.4621) (-0.2933, 21.398) (-0.3029, 21.3339) (-0.3105, 21.2697) (-0.3142, 21.2182) (-0.3153, 21.1795) (-0.3153, 21.1537) (-0.3151, 21.1407) knots -1 -1 -1 -1 -1 -1 -0.98571429 -0.97142857 -0.95714286 -0.94285714 -0.92857143 -0.91428571 -0.9 -0.88571429 -0.87142857 -0.85714286 -0.84285714 -0.82857143 -0.81428571 -0.8 -0.78571429 -0.77142857 -0.75714286 -0.74285714 -0.72857143 -0.71428571 -0.7 -0.68571429 -0.67142857 -0.65714286 -0.64285714 -0.62857143 -0.61428571 -0.6 -0.58571429 -0.57142857 -0.55714286 -0.54285714 -0.52857143 -0.51428571 -0.5 -0.48571429 -0.47142857 -0.45714286 -0.44285714 -0.42857143 -0.41428571 -0.4 -0.38571429 -0.37142857 -0.35714286 -0.34285714 -0.32857143 -0.31428571 -0.3 -0.28571429 -0.27142857 -0.25714286 -0.24285714 -0.22857143 -0.21428571 -0.2 -0.18571429 -0.17142857 -0.15714286 -0.14285714 -0.12857143 -0.11428571 -0.1 -0.08571429 -0.07142857 -0.05714286 -0.04285714 -0.02857143 -0.01428571 0 0 0 0 0 0
  line L23 (-0.3151, 21.1407) -> (-0.3029, 20.2908)
  arc A47 (-1.6698, 18.7751) -> (-0.3029, 20.2908) centre (-1.8027, 20.2692) ccw
  arc A48 (-1.6698, 18.7751) -> (-2.2702, 18.712) centre (0, 0) ccw
  arc A49 (-3.9224, 19.9103) -> (-2.2702, 18.712) centre (-2.4509, 20.2011) ccw
  line L24 (-3.9224, 19.9103) -> (-4.0872, 20.7443)
  spline S24 degree 5 poles (-4.0872, 20.7443) (-4.0897, 20.757) (-4.0951, 20.7822) (-4.1042, 20.8198) (-4.1185, 20.8694) (-4.1392, 20.9307) (-4.162, 20.9914) (-4.186, 21.0518) (-4.2108, 21.1121) (-4.236, 21.1722) (-4.2617, 21.2322) (-4.288, 21.292) (-4.3153, 21.3515) (-4.3435, 21.4108) (-4.3727, 21.4698) (-4.4028, 21.5285) (-4.4337, 21.5869) (-4.4653, 21.6451) (-4.4974, 21.7031) (-4.5301, 21.761) (-4.5633, 21.8187) (-4.5971, 21.8761) (-4.6316, 21.9334) (-4.6666, 21.9904) (-4.7022, 22.0472) (-4.7384, 22.1038) (-4.7752, 22.1602) (-4.8125, 22.2164) (-4.8503, 22.2724) (-4.8886, 22.3282) (-4.9273, 22.3838) (-4.9666, 22.4392) (-5.0064, 22.4944) (-5.0466, 22.5494) (-5.0874, 22.6043) (-5.1286, 22.6589) (-5.1702, 22.7133) (-5.2124, 22.7675) (-5.2549, 22.8215) (-5.2979, 22.8753) (-5.3414, 22.9289) (-5.3853, 22.9824) (-5.4296, 23.0356) (-5.4743, 23.0886) (-5.5194, 23.1414) (-5.565, 23.194) (-5.611, 23.2465) (-5.6573, 23.2987) (-5.7041, 23.3507) (-5.7513, 23.4025) (-5.7988, 23.4541) (-5.8468, 23.5056) (-5.8951, 23.5568) (-5.9438, 23.6078) (-5.9929, 23.6586) (-6.0424, 23.7092) (-6.0922, 23.7596) (-6.1425, 23.8098) (-6.193, 23.8598) (-6.244, 23.9096) (-6.2953, 23.9592) (-6.3469, 24.0086) (-6.3989, 24.0578) (-6.4513, 24.1067) (-6.504, 24.1555) (-6.557, 24.2041) (-6.6104, 24.2524) (-6.6642, 24.3005) (-6.7182, 24.3485) (-6.7726, 24.3962) (-6.8274, 24.4437) (-6.8714, 24.4815) (-6.9046, 24.5098) (-6.9268, 24.5286) (-6.9379, 24.538) knots 0 0 0 0 0 0 0.01428571 0.02857143 0.04285714 0.05714286 0.07142857 0.08571429 0.1 0.11428571 0.12857143 0.14285714 0.15714286 0.17142857 0.18571429 0.2 0.21428571 0.22857143 0.24285714 0.25714286 0.27142857 0.28571429 0.3 0.31428571 0.32857143 0.34285714 0.35714286 0.37142857 0.38571429 0.4 0.41428571 0.42857143 0.44285714 0.45714286 0.47142857 0.48571429 0.5 0.51428571 0.52857143 0.54285714 0.55714286 0.57142857 0.58571429 0.6 0.61428571 0.62857143 0.64285714 0.65714286 0.67142857 0.68571429 0.7 0.71428571 0.72857143 0.74285714 0.75714286 0.77142857 0.78571429 0.8 0.81428571 0.82857143 0.84285714 0.85714286 0.87142857 0.88571429 0.9 0.91428571 0.92857143 0.94285714 0.95714286 0.97142857 0.98571429 1 1 1 1 1 1
  arc A50 (-6.9379, 24.538) -> (-8.8102, 23.9297) centre (0, 0) ccw
  spline S25 degree 5 poles (-8.8102, 23.9297) (-8.8137, 23.9156) (-8.8206, 23.8873) (-8.8308, 23.8449) (-8.8442, 23.7884) (-8.8606, 23.7178) (-8.8765, 23.6472) (-8.8921, 23.5766) (-8.9073, 23.5061) (-8.922, 23.4356) (-8.9364, 23.3652) (-8.9504, 23.2947) (-8.964, 23.2243) (-8.9771, 23.154) (-8.9899, 23.0837) (-9.0022, 23.0134) (-9.0142, 22.9432) (-9.0257, 22.873) (-9.0368, 22.8029) (-9.0475, 22.7328) (-9.0578, 22.6628) (-9.0676, 22.5928) (-9.0771, 22.5229) (-9.0861, 22.453) (-9.0946, 22.3833) (-9.1028, 22.3135) (-9.1105, 22.2439) (-9.1177, 22.1743) (-9.1246, 22.1048) (-9.1309, 22.0354) (-9.1369, 21.966) (-9.1423, 21.8968) (-9.1474, 21.8276) (-9.1519, 21.7585) (-9.156, 21.6895) (-9.1596, 21.6206) (-9.1628, 21.5518) (-9.1655, 21.483) (-9.1677, 21.4144) (-9.1694, 21.3459) (-9.1707, 21.2775) (-9.1714, 21.2092) (-9.1717, 21.1411) (-9.1714, 21.073) (-9.1706, 21.0051) (-9.1693, 20.9373) (-9.1674, 20.8697) (-9.1651, 20.8022) (-9.1622, 20.7348) (-9.1588, 20.6675) (-9.1549, 20.6005) (-9.1503, 20.5335) (-9.1451, 20.4668) (-9.1393, 20.4003) (-9.1329, 20.3339) (-9.1258, 20.2678) (-9.1183, 20.2017) (-9.1102, 20.1359) (-9.1015, 20.0702) (-9.0922, 20.0048) (-9.082, 19.9396) (-9.071, 19.8747) (-9.059, 19.8102) (-9.046, 19.746) (-9.0322, 19.6821) (-9.0177, 19.6185) (-9.0028, 19.555) (-8.9874, 19.4918) (-8.9713, 19.4288) (-8.954, 19.3663) (-8.9348, 19.3045) (-8.9172, 19.256) (-8.9025, 19.2202) (-8.892, 19.1966) (-8.8866, 19.1849) knots -1 -1 -1 -1 -1 -1 -0.98571429 -0.97142857 -0.95714286 -0.94285714 -0.92857143 -0.91428571 -0.9 -0.88571429 -0.87142857 -0.85714286 -0.84285714 -0.82857143 -0.81428571 -0.8 -0.78571429 -0.77142857 -0.75714286 -0.74285714 -0.72857143 -0.71428571 -0.7 -0.68571429 -0.67142857 -0.65714286 -0.64285714 -0.62857143 -0.61428571 -0.6 -0.58571429 -0.57142857 -0.55714286 -0.54285714 -0.52857143 -0.51428571 -0.5 -0.48571429 -0.47142857 -0.45714286 -0.44285714 -0.42857143 -0.41428571 -0.4 -0.38571429 -0.37142857 -0.35714286 -0.34285714 -0.32857143 -0.31428571 -0.3 -0.28571429 -0.27142857 -0.25714286 -0.24285714 -0.22857143 -0.21428571 -0.2 -0.18571429 -0.17142857 -0.15714286 -0.14285714 -0.12857143 -0.11428571 -0.1 -0.08571429 -0.07142857 -0.05714286 -0.04285714 -0.02857143 -0.01428571 0 0 0 0 0 0
  line L25 (-8.8866, 19.1849) -> (-8.5297, 18.4134)
  arc A51 (-9.162, 16.4727) -> (-8.5297, 18.4134) centre (-9.8911, 17.7836) ccw
  arc A52 (-9.162, 16.4727) -> (-9.6848, 16.1709) centre (0, 0) ccw
  arc A53 (-11.6816, 16.5936) -> (-9.6848, 16.1709) centre (-10.4555, 17.4577) ccw
  line L26 (-11.6816, 16.5936) -> (-12.1713, 17.2884)
  spline S26 degree 5 poles (-12.1713, 17.2884) (-12.1787, 17.299) (-12.1939, 17.3199) (-12.2176, 17.3505) (-12.2508, 17.39) (-12.2947, 17.4376) (-12.3402, 17.4838) (-12.3867, 17.5292) (-12.4338, 17.5742) (-12.4813, 17.6188) (-12.5291, 17.6632) (-12.5775, 17.7071) (-12.6266, 17.7504) (-12.6765, 17.7931) (-12.7272, 17.8351) (-12.7786, 17.8764) (-12.8306, 17.9172) (-12.8831, 17.9576) (-12.9361, 17.9975) (-12.9895, 18.0371) (-13.0433, 18.0763) (-13.0975, 18.115) (-13.1522, 18.1533) (-13.2074, 18.1912) (-13.2631, 18.2286) (-13.3192, 18.2656) (-13.3757, 18.3021) (-13.4326, 18.3383) (-13.4899, 18.3741) (-13.5476, 18.4095) (-13.6057, 18.4445) (-13.6641, 18.4792) (-13.7229, 18.5134) (-13.782, 18.5473) (-13.8415, 18.5808) (-13.9014, 18.6139) (-13.9616, 18.6467) (-14.0221, 18.6791) (-14.083, 18.7111) (-14.1441, 18.7428) (-14.2056, 18.7741) (-14.2674, 18.805) (-14.3296, 18.8356) (-14.392, 18.8659) (-14.4547, 18.8958) (-14.5177, 18.9253) (-14.5811, 18.9545) (-14.6447, 18.9834) (-14.7085, 19.0119) (-14.7727, 19.04) (-14.8372, 19.0678) (-14.9019, 19.0953) (-14.9669, 19.1224) (-15.0321, 19.1492) (-15.0976, 19.1757) (-15.1634, 19.2018) (-15.2295, 19.2276) (-15.2957, 19.253) (-15.3623, 19.2781) (-15.4291, 19.3029) (-15.4961, 19.3273) (-15.5634, 19.3514) (-15.6309, 19.3752) (-15.6986, 19.3986) (-15.7666, 19.4217) (-15.8348, 19.4445) (-15.9033, 19.467) (-15.9719, 19.4891) (-16.0408, 19.5109) (-16.1099, 19.5324) (-16.1792, 19.5535) (-16.2349, 19.5702) (-16.2767, 19.5825) (-16.3046, 19.5907) (-16.3186, 19.5947) knots 0 0 0 0 0 0 0.01428571 0.02857143 0.04285714 0.05714286 0.07142857 0.08571429 0.1 0.11428571 0.12857143 0.14285714 0.15714286 0.17142857 0.18571429 0.2 0.21428571 0.22857143 0.24285714 0.25714286 0.27142857 0.28571429 0.3 0.31428571 0.32857143 0.34285714 0.35714286 0.37142857 0.38571429 0.4 0.41428571 0.42857143 0.44285714 0.45714286 0.47142857 0.48571429 0.5 0.51428571 0.52857143 0.54285714 0.55714286 0.57142857 0.58571429 0.6 0.61428571 0.62857143 0.64285714 0.65714286 0.67142857 0.68571429 0.7 0.71428571 0.72857143 0.74285714 0.75714286 0.77142857 0.78571429 0.8 0.81428571 0.82857143 0.84285714 0.85714286 0.87142857 0.88571429 0.9 0.91428571 0.92857143 0.94285714 0.95714286 0.97142857 0.98571429 1 1 1 1 1 1
  arc A54 (-16.3186, 19.5947) -> (-17.7816, 18.2774) centre (0, 0) ccw
  spline S27 degree 5 poles (-17.7816, 18.2774) (-17.779, 18.2631) (-17.7738, 18.2345) (-17.7659, 18.1916) (-17.7552, 18.1345) (-17.7414, 18.0634) (-17.7273, 17.9924) (-17.7128, 17.9216) (-17.698, 17.851) (-17.6828, 17.7806) (-17.6673, 17.7104) (-17.6514, 17.6403) (-17.6352, 17.5705) (-17.6186, 17.5009) (-17.6016, 17.4315) (-17.5843, 17.3622) (-17.5667, 17.2932) (-17.5487, 17.2244) (-17.5303, 17.1558) (-17.5116, 17.0875) (-17.4925, 17.0193) (-17.473, 16.9514) (-17.4532, 16.8837) (-17.433, 16.8162) (-17.4125, 16.749) (-17.3915, 16.682) (-17.3702, 16.6152) (-17.3486, 16.5487) (-17.3265, 16.4825) (-17.3041, 16.4164) (-17.2813, 16.3507) (-17.2582, 16.2852) (-17.2346, 16.2199) (-17.2107, 16.1549) (-17.1863, 16.0902) (-17.1616, 16.0258) (-17.1365, 15.9617) (-17.111, 15.8978) (-17.0852, 15.8342) (-17.0589, 15.7709) (-17.0322, 15.7079) (-17.0051, 15.6452) (-16.9776, 15.5829) (-16.9496, 15.5208) (-16.9213, 15.4591) (-16.8925, 15.3977) (-16.8633, 15.3367) (-16.8337, 15.2759) (-16.8037, 15.2155) (-16.7733, 15.1555) (-16.7423, 15.0958) (-16.711, 15.0366) (-16.6791, 14.9777) (-16.6467, 14.9193) (-16.6138, 14.8613) (-16.5805, 14.8037) (-16.5468, 14.7465) (-16.5126, 14.6896) (-16.4779, 14.6332) (-16.4428, 14.5772) (-16.407, 14.5217) (-16.3706, 14.467) (-16.3334, 14.4129) (-16.2954, 14.3595) (-16.2568, 14.3068) (-16.2177, 14.2546) (-16.1782, 14.2027) (-16.1384, 14.1511) (-16.0981, 14.1001) (-16.0569, 14.05) (-16.0142, 14.0015) (-15.9784, 13.9643) (-15.9504, 13.9375) (-15.9312, 13.9202) (-15.9215, 13.9117) knots -1 -1 -1 -1 -1 -1 -0.98571429 -0.97142857 -0.95714286 -0.94285714 -0.92857143 -0.91428571 -0.9 -0.88571429 -0.87142857 -0.85714286 -0.84285714 -0.82857143 -0.81428571 -0.8 -0.78571429 -0.77142857 -0.75714286 -0.74285714 -0.72857143 -0.71428571 -0.7 -0.68571429 -0.67142857 -0.65714286 -0.64285714 -0.62857143 -0.61428571 -0.6 -0.58571429 -0.57142857 -0.55714286 -0.54285714 -0.52857143 -0.51428571 -0.5 -0.48571429 -0.47142857 -0.45714286 -0.44285714 -0.42857143 -0.41428571 -0.4 -0.38571429 -0.37142857 -0.35714286 -0.34285714 -0.32857143 -0.31428571 -0.3 -0.28571429 -0.27142857 -0.25714286 -0.24285714 -0.22857143 -0.21428571 -0.2 -0.18571429 -0.17142857 -0.15714286 -0.14285714 -0.12857143 -0.11428571 -0.1 -0.08571429 -0.07142857 -0.05714286 -0.04285714 -0.02857143 -0.01428571 0 0 0 0 0 0
  line L27 (-15.9215, 13.9117) -> (-15.2817, 13.3521)
  arc A55 (-15.07, 11.3221) -> (-15.2817, 13.3521) centre (-16.2692, 12.223) ccw
  arc A56 (-15.07, 11.3221) -> (-15.4248, 10.8337) centre (0, 0) ccw
  arc A57 (-17.4209, 10.4077) -> (-15.4248, 10.8337) centre (-16.6523, 11.6958) ccw
  line L28 (-17.4209, 10.4077) -> (-18.1509, 10.8433)
  spline S28 degree 5 poles (-18.1509, 10.8433) (-18.162, 10.8499) (-18.1843, 10.8628) (-18.2184, 10.8812) (-18.2648, 10.9037) (-18.3242, 10.9293) (-18.3846, 10.953) (-18.4456, 10.9756) (-18.5069, 10.9975) (-18.5684, 11.019) (-18.6302, 11.0401) (-18.6923, 11.0605) (-18.7548, 11.0801) (-18.8177, 11.0988) (-18.881, 11.1165) (-18.9448, 11.1334) (-19.0089, 11.1495) (-19.0733, 11.165) (-19.138, 11.18) (-19.2028, 11.1944) (-19.2679, 11.2083) (-19.3332, 11.2216) (-19.3988, 11.2344) (-19.4646, 11.2465) (-19.5307, 11.258) (-19.597, 11.269) (-19.6635, 11.2794) (-19.7302, 11.2893) (-19.7971, 11.2987) (-19.8642, 11.3076) (-19.9315, 11.316) (-19.9989, 11.3239) (-20.0665, 11.3313) (-20.1344, 11.3381) (-20.2023, 11.3446) (-20.2705, 11.3505) (-20.3388, 11.3559) (-20.4073, 11.3609) (-20.4759, 11.3654) (-20.5447, 11.3694) (-20.6136, 11.373) (-20.6827, 11.3762) (-20.7518, 11.3789) (-20.8212, 11.3811) (-20.8906, 11.3829) (-20.9602, 11.3842) (-21.0299, 11.3852) (-21.0998, 11.3856) (-21.1697, 11.3857) (-21.2398, 11.3853) (-21.31, 11.3845) (-21.3803, 11.3833) (-21.4507, 11.3816) (-21.5212, 11.3796) (-21.5918, 11.3771) (-21.6625, 11.3742) (-21.7333, 11.3709) (-21.8043, 11.3671) (-21.8752, 11.363) (-21.9463, 11.3585) (-22.0175, 11.3535) (-22.0888, 11.3482) (-22.1601, 11.3425) (-22.2315, 11.3363) (-22.303, 11.3298) (-22.3746, 11.3228) (-22.4463, 11.3155) (-22.518, 11.3078) (-22.5898, 11.2997) (-22.6617, 11.2912) (-22.7336, 11.2823) (-22.7912, 11.2749) (-22.8344, 11.2692) (-22.8633, 11.2653) (-22.8777, 11.2633) knots 0 0 0 0 0 0 0.01428571 0.02857143 0.04285714 0.05714286 0.07142857 0.08571429 0.1 0.11428571 0.12857143 0.14285714 0.15714286 0.17142857 0.18571429 0.2 0.21428571 0.22857143 0.24285714 0.25714286 0.27142857 0.28571429 0.3 0.31428571 0.32857143 0.34285714 0.35714286 0.37142857 0.38571429 0.4 0.41428571 0.42857143 0.44285714 0.45714286 0.47142857 0.48571429 0.5 0.51428571 0.52857143 0.54285714 0.55714286 0.57142857 0.58571429 0.6 0.61428571 0.62857143 0.64285714 0.65714286 0.67142857 0.68571429 0.7 0.71428571 0.72857143 0.74285714 0.75714286 0.77142857 0.78571429 0.8 0.81428571 0.82857143 0.84285714 0.85714286 0.87142857 0.88571429 0.9 0.91428571 0.92857143 0.94285714 0.95714286 0.97142857 0.98571429 1 1 1 1 1 1
  arc A58 (-22.8777, 11.2633) -> (-23.6784, 9.4648) centre (0, 0) ccw
  spline S29 degree 5 poles (-23.6784, 9.4648) (-23.6702, 9.4528) (-23.6538, 9.4287) (-23.6292, 9.3928) (-23.5961, 9.345) (-23.5546, 9.2856) (-23.5128, 9.2265) (-23.4708, 9.1677) (-23.4286, 9.1093) (-23.3861, 9.0511) (-23.3433, 8.9933) (-23.3003, 8.9358) (-23.2571, 8.8786) (-23.2136, 8.8217) (-23.1699, 8.7652) (-23.126, 8.709) (-23.0818, 8.6531) (-23.0373, 8.5976) (-22.9926, 8.5424) (-22.9477, 8.4876) (-22.9026, 8.4331) (-22.8572, 8.379) (-22.8115, 8.3252) (-22.7656, 8.2718) (-22.7195, 8.2187) (-22.6731, 8.166) (-22.6265, 8.1137) (-22.5797, 8.0617) (-22.5326, 8.0101) (-22.4853, 7.9589) (-22.4377, 7.9081) (-22.3899, 7.8577) (-22.3418, 7.8077) (-22.2935, 7.7581) (-22.245, 7.7088) (-22.1962, 7.66) (-22.1472, 7.6116) (-22.0979, 7.5637) (-22.0484, 7.5161) (-21.9987, 7.469) (-21.9487, 7.4223) (-21.8984, 7.376) (-21.8479, 7.3303) (-21.7972, 7.2849) (-21.7462, 7.2401) (-21.6949, 7.1957) (-21.6434, 7.1518) (-21.5917, 7.1084) (-21.5397, 7.0654) (-21.4874, 7.0229) (-21.4349, 6.981) (-21.3821, 6.9396) (-21.3291, 6.8988) (-21.2757, 6.8586) (-21.2221, 6.819) (-21.1683, 6.7799) (-21.1141, 6.7414) (-21.0598, 6.7034) (-21.0052, 6.6659) (-20.9503, 6.629) (-20.8951, 6.5929) (-20.8395, 6.5577) (-20.7835, 6.5235) (-20.7271, 6.4902) (-20.6704, 6.4577) (-20.6134, 6.4259) (-20.5563, 6.3945) (-20.4989, 6.3636) (-20.4414, 6.3334) (-20.3834, 6.3044) (-20.3246, 6.2774) (-20.2768, 6.258) (-20.2403, 6.245) (-20.2158, 6.237) (-20.2034, 6.2332) knots -1 -1 -1 -1 -1 -1 -0.98571429 -0.97142857 -0.95714286 -0.94285714 -0.92857143 -0.91428571 -0.9 -0.88571429 -0.87142857 -0.85714286 -0.84285714 -0.82857143 -0.81428571 -0.8 -0.78571429 -0.77142857 -0.75714286 -0.74285714 -0.72857143 -0.71428571 -0.7 -0.68571429 -0.67142857 -0.65714286 -0.64285714 -0.62857143 -0.61428571 -0.6 -0.58571429 -0.57142857 -0.55714286 -0.54285714 -0.52857143 -0.51428571 -0.5 -0.48571429 -0.47142857 -0.45714286 -0.44285714 -0.42857143 -0.41428571 -0.4 -0.38571429 -0.37142857 -0.35714286 -0.34285714 -0.32857143 -0.31428571 -0.3 -0.28571429 -0.27142857 -0.25714286 -0.24285714 -0.22857143 -0.21428571 -0.2 -0.18571429 -0.17142857 -0.15714286 -0.14285714 -0.12857143 -0.11428571 -0.1 -0.08571429 -0.07142857 -0.05714286 -0.04285714 -0.02857143 -0.01428571 0 0 0 0 0 0
  line L29 (-20.2034, 6.2332) -> (-19.3913, 5.9821)
  arc A59 (-18.3722, 4.2137) -> (-19.3913, 5.9821) centre (-19.8342, 4.549) ccw
  circle A60 centre (0, 0) radius 4
  circle A61 centre (0, 0) radius 5
  circle A62 centre (0, 0) radius 7.5
  dimension "d159" = 10
  dimension "d160" = 15
  constraint concentric A0 A61
  constraint concentric A0 A62
  measures "d159" diameter of A61
  measures "d160" diameter of A62
extrude "Extrude3'''" add sketch "Sketch4 (3)" along normal blind 5 contours A62 bodies 4 in component "Spur Gear (15 teeth) (1)"